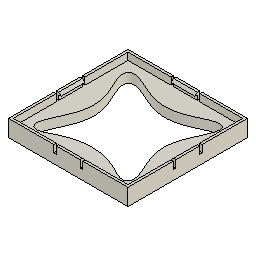
halterPlatinen v6 (Autodesk Fusion 360 design; units mm, degrees)
Autodesk Fusion 360 part; units mm, degrees
sketch "Skizze1" plane through (0, 0, 0) normal (0, 0, 1) x (1, 0, 0)
  line L0 (25, 25) -> (-25, 25)
  line L1 (-25, 25) -> (-25, -25)
  line L2 (-25, -25) -> (25, -25)
  line L3 (25, -25) -> (25, 25)
  line L4 (25, 25) -> (-25, -25) construction
  line L5 (-25, 25) -> (25, -25) construction
  line L6 (0, 25) -> (0, 21.5) construction
  circle A0 centre (0, 21.5) radius 2.5
  circle A1 centre (-21.5, 0) radius 2.5
  circle A2 centre (0, -21.5) radius 2.5
  circle A3 centre (21.5, 0) radius 2.5
  line L7 (-25, 25) -> (-19.6967, 19.6967)
  line L8 (25, 25) -> (19.6967, 19.6967)
  line L9 (25, -25) -> (19.6967, -19.6967)
  line L10 (-25, -25) -> (-19.6967, -19.6967)
  line L11 (0, 25) -> (0, 15) construction
  line L12 (25, 0) -> (15, 0) construction
  line L13 (0, -25) -> (0, -15) construction
  line L14 (-25, 0) -> (-15, 0) construction
  spline S0 degree 5 poles (0, -15) (1.2065, -15) (3.6254, -15.1465) (7.1572, -15.8132) (11.2047, -17.4413) (15.1309, -19.6326) (18.0012, -20.8352) (20.0511, -20.1301) (20.6752, -17.6735) (19.5115, -14.1604) (17.3962, -9.8731) (15.4021, -5.0946) (14.5897, -0.0184) (15.4512, 5.1337) (17.4986, 10.0731) (19.6685, 14.4705) (20.838, 17.9349) (20.126, 20.1337) (17.6793, 20.5662) (14.1665, 19.2783) (9.8729, 17.155) (5.088, 15.2723) (0.0153, 14.6011) (-5.1205, 15.5565) (-10.0405, 17.6249) (-14.4307, 19.7595) (-17.9076, 20.8718) (-20.1386, 20.1183) (-20.5833, 17.6619) (-19.2644, 14.1613) (-17.1004, 9.8864) (-15.2073, 5.1088) (-14.5882, 0.0204) (-15.6493, -5.152) (-17.8106, -10.1075) (-19.9406, -14.5038) (-20.9509, -17.9505) (-20.0386, -20.1219) (-17.7519, -20.5757) (-14.8416, -19.3727) (-11.0208, -17.3175) (-7.0919, -15.7983) (-3.6135, -15.1465) (-1.2065, -15) (0, -15) knots 0 0 0 0 0 0 0.025 0.05 0.075 0.1 0.125 0.15 0.175 0.2 0.225 0.25 0.275 0.3 0.325 0.35 0.375 0.4 0.425 0.45 0.475 0.5 0.525 0.55 0.575 0.6 0.625 0.65 0.675 0.7 0.725 0.75 0.775 0.8 0.825 0.85 0.875 0.9 0.925 0.95 0.975 1 1 1 1 1 1
  line L15 (-21.5565, -18.1362) -> (-17.8369, -21.2572)
  line L16 (-8.8743, -15) -> (8.8743, -15)
  line L17 (21.5565, 18.1362) -> (17.8369, 21.2572)
  line L18 (18.1362, -21.5565) -> (21.2572, -17.8369)
  line L19 (-18.1127, 21.5869) -> (-21.2807, 17.8065)
  line L20 (2.5, 19) -> (-2.5, 19)
  line L21 (-2.5, 19) -> (-2.5, 24)
  line L22 (-2.5, 24) -> (2.5, 24)
  line L23 (2.5, 24) -> (2.5, 19)
  line L24 (2.5, 19) -> (-2.5, 24) construction
  line L25 (-2.5, 19) -> (2.5, 24) construction
  line L26 (-19, 2.5) -> (-19, -2.5)
  line L27 (-24, 2.5) -> (-19, 2.5)
  line L28 (-24, -2.5) -> (-24, 2.5)
  line L29 (-19, -2.5) -> (-24, -2.5)
  line L30 (-2.5, -19) -> (2.5, -19)
  line L31 (-2.5, -24) -> (-2.5, -19)
  line L32 (2.5, -24) -> (-2.5, -24)
  line L33 (2.5, -19) -> (2.5, -24)
  line L34 (19, -2.5) -> (19, 2.5)
  line L35 (24, -2.5) -> (19, -2.5)
  line L36 (24, 2.5) -> (24, -2.5)
  line L37 (19, 2.5) -> (24, 2.5)
  point P0 (0, 21.5)
  dimension "d1" = 50
  dimension "d2" = 50
  dimension "d4" = 5
  dimension "d6" = 360
  dimension "d7" = 7.5
  dimension "d8" = 7.5
  dimension "d9" = 7.5
  dimension "d10" = 7.5
  dimension "d11" = 10
  dimension "d12" = 10
  dimension "d13" = 10
  dimension "d14" = 10
  dimension "d39" = 5
  dimension "d40" = 5
  dimension "d42" = 360
  dimension "d43" = 3.5
  constraint perpendicular L0 L1
  constraint parallel L0 L2
  constraint parallel L1 L3
  constraint horizontal L0
  constraint coincident L4 origin
  constraint coincident L5 origin
  constraint midpoint L0 L6.start
  constraint perpendicular L0 L6
  constraint coincident P0 L6.end
  constraint parallel L5 L7
  constraint parallel L4 L8
  constraint parallel L5 L9
  constraint parallel L4 L10
  constraint perpendicular L0 L11
  constraint midpoint L3 L12.start
  constraint perpendicular L3 L12
  constraint midpoint L2 L13.start
  constraint perpendicular L2 L13
  constraint midpoint L1 L14.start
  constraint perpendicular L1 L14
  constraint midpoint L10.end L15
  constraint midpoint L13.end L16
  constraint midpoint L8.end L17
  constraint midpoint L9.end L18
  constraint midpoint L7.end L19
  constraint perpendicular L20 L21
  constraint parallel L20 L22
  constraint parallel L21 L23
  constraint horizontal L20
  constraint coincident L24 P0
  constraint coincident L25 P0
  measures "d1" distance of L1.end L2.end
  measures "d2" distance of L0.end L1.end
  measures "d4" diameter of A0
  measures "d7" distance of L0.end L7.end
  measures "d8" distance of L0.start L8.end
  measures "d9" distance of L2.end L9.end
  measures "d10" distance of L1.end L10.end
  measures "d11" distance of L6.start L11.end
  measures "d12" distance of L12.start L12.end
  measures "d13" distance of L13.start L13.end
  measures "d14" distance of L14.start L14.end
  measures "d39" distance of L20.end L21.end
  measures "d40" distance of L21.end L22.end
  measures "d43" distance of L6.start P0
extrude "Extrusion1" add sketch "Skizze1" along normal blind 4 contours L0 L7 L8 S0 | L3 L8 L9 S0 | L1 L7 L10 S0 | L2 L9 L10 S0 | A0 | A0 L20 L23 | A0 L22 L23 | A0 L21 L22 | A0 L20 L21 | A1 | A1 L26 L29 | A1 L26 L27 | A1 L27 L28 | A1 L28 L29 | A2 | A2 L32 L33 | A2 L30 L33 | A2 L30 L31 | A2 L31 L32 | A3 | A3 L35 L36 | A3 L36 L37 | A3 L34 L37 | A3 L34 L35
sketch "Skizze9" plane through (0, 0, 4) normal (0, 0, 1) x (-1, 0, 0)
  spline S0 degree 5 poles (0, 15) (1.2065, 15) (3.6135, 15.1465) (7.0919, 15.7983) (11.0208, 17.3175) (14.8416, 19.3727) (17.7519, 20.5757) (20.0386, 20.1219) (20.9509, 17.9505) (19.9406, 14.5038) (17.8106, 10.1075) (15.6493, 5.152) (14.5882, -0.0204) (15.2073, -5.1088) (17.1004, -9.8864) (19.2644, -14.1613) (20.5833, -17.6619) (20.1386, -20.1183) (17.9076, -20.8718) (14.4307, -19.7595) (10.0405, -17.6249) (5.1205, -15.5565) (-0.0153, -14.6011) (-5.088, -15.2723) (-9.8729, -17.155) (-14.1665, -19.2783) (-17.6793, -20.5662) (-20.126, -20.1337) (-20.838, -17.9349) (-19.6685, -14.4705) (-17.4986, -10.0731) (-15.4512, -5.1337) (-14.5897, 0.0184) (-15.4021, 5.0946) (-17.3962, 9.8731) (-19.5115, 14.1604) (-20.6752, 17.6735) (-20.0511, 20.1301) (-18.0012, 20.8352) (-15.1309, 19.6326) (-11.2047, 17.4413) (-7.1572, 15.8132) (-3.6254, 15.1465) (-1.2065, 15) (0, 15) knots -1 -1 -1 -1 -1 -1 -0.975 -0.95 -0.925 -0.9 -0.875 -0.85 -0.825 -0.8 -0.775 -0.75 -0.725 -0.7 -0.675 -0.65 -0.625 -0.6 -0.575 -0.55 -0.525 -0.5 -0.475 -0.45 -0.425 -0.4 -0.375 -0.35 -0.325 -0.3 -0.275 -0.25 -0.225 -0.2 -0.175 -0.15 -0.125 -0.1 -0.075 -0.05 -0.025 0 0 0 0 0 0
  line L0 (-25, 25) -> (-25, -25)
  line L1 (-25, -25) -> (25, -25)
  line L2 (25, -25) -> (25, 25)
  line L3 (25, 25) -> (-25, 25)
  line L4 (24, 24) -> (-24, 24)
  line L5 (-24, 24) -> (-24, -24)
  line L6 (-24, -24) -> (24, -24)
  line L7 (24, -24) -> (24, 24)
  line L8 (0, -25) -> (-5, -25)
  line L9 (-5, -25) -> (-5, -24)
  line L10 (-5, -25) -> (-6, -25)
  line L11 (-6, -25) -> (-6, -24)
  line L12 (0, -25) -> (0, -24) construction
  line L13 (6, -25) -> (6, -24)
  line L14 (5, -25) -> (5, -24)
  line L15 (5, -24) -> (-5, -24)
  line L16 (-5, -24) -> (-5, -23)
  line L17 (-5, -23) -> (5, -23)
  line L18 (5, -23) -> (5, -24)
  line L19 (25, 6) -> (24, 6)
  line L20 (25, 5) -> (24, 5)
  line L21 (23, 5) -> (24, 5)
  line L22 (23, -5) -> (23, 5)
  line L23 (25, -5) -> (24, -5)
  line L24 (25, -6) -> (24, -6)
  line L25 (24, -5) -> (23, -5)
  line L26 (-6, 25) -> (-6, 24)
  line L27 (-5, 25) -> (-5, 24)
  line L28 (-5, 23) -> (-5, 24)
  line L29 (5, 23) -> (-5, 23)
  line L30 (5, 25) -> (5, 24)
  line L31 (6, 25) -> (6, 24)
  line L32 (5, 24) -> (5, 23)
  line L33 (-25, -6) -> (-24, -6)
  line L34 (-25, -5) -> (-24, -5)
  line L35 (-23, -5) -> (-24, -5)
  line L36 (-23, 5) -> (-23, -5)
  line L37 (-25, 5) -> (-24, 5)
  line L38 (-25, 6) -> (-24, 6)
  line L39 (-24, 5) -> (-23, 5)
  dimension "d65" = -1
  dimension "d66" = 5
  dimension "d67" = 1
  dimension "d70" = 0
  dimension "d71" = 0
  dimension "d72" = 10
  dimension "d73" = 1
  dimension "d75" = 360
  constraint midpoint L1 L8.start
  constraint parallel L1 L8
  constraint coincident L6 L9.end
  constraint perpendicular L6 L9
  constraint perpendicular L9 L10
  constraint coincident L6 L11.end
  constraint perpendicular L6 L11
  constraint midpoint L6 L12.end
  constraint symmetric L8.end L12 L14.start
  constraint symmetric L9.end L12 L14.end
  constraint symmetric L10.end L12 L13.start
  constraint symmetric L11.end L12 L13.end
  constraint horizontal L15
  constraint vertical L16
  constraint horizontal L17
  constraint vertical L18
  measures "d66" distance of L8.start L8.end
  measures "d67" distance of L8.end L10.end
  measures "d72" distance of L14.end L9.end
  measures "d73" distance of L14.end L17.end
extrude "Extrusion12" add sketch "Skizze9" along normal blind 3 contours L0 L3 L4 L5 L26 L38 | L0 L5 L34 L37 | L3 L4 L27 L30 | L5 L35 L36 L39 | L4 L28 L29 L32 | L0 L1 L5 L6 L11 L33 | L2 L3 L4 L7 L19 L31 | L1 L6 L8 L9 L14 L15 | L2 L7 L20 L23 | L6 L15 L16 L17 L18 | L7 L21 L22 L25 | L1 L2 L6 L7 L13 L24
extrude "Extrusion13" cut sketch "Skizze9" along normal blind 2 contours L5 L35 L36 L39 | L4 L28 L29 L32 | L6 L15 L16 L17 L18 | L7 L21 L22 L25
chamfer "Fase1" distance 1 angle 45 4 edges at (23, 0, 7) (0, -23, 7) (-23, 0, 7) (0, 23, 7)
extrude "Extrusion14" cut sketch "Skizze1" along normal blind 2.5 contours A0 | A0 L20 L23 | A0 L22 L23 | A0 L21 L22 | A0 L20 L21 | A1 | A1 L26 L29 | A1 L26 L27 | A1 L27 L28 | A1 L28 L29 | A2 | A2 L32 L33 | A2 L30 L33 | A2 L30 L31 | A2 L31 L32 | A3 | A3 L35 L36 | A3 L36 L37 | A3 L34 L37 | A3 L34 L35
named bodies: "Top"
